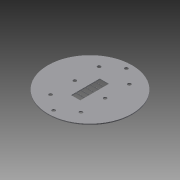
# Autodesk Inventor part: Plate
Saved by Autodesk Inventor 2013 (Build 170138000, 138)
## iProperties
Created: 2014-03-14
Part Number: Plate
Material: Generic
Document SubType Name: Sheet Metal
Designer: jad211
Density: 1 g/cm^3
Sheet Metal Rule: Default_mm
Author: jad211
Autodesk Inventor part; units mm, degrees
ref_plane "YZ Plane" through (0, 0, 0) normal (1, 0, 0) x (0, 1, 0)
ref_plane "XZ Plane" through (0, 0, 0) normal (0, 1, 0) x (-1, 0, 0)
ref_plane "XY Plane" through (0, 0, 0) normal (0, 0, 1) x (1, 0, 0)
sketch "Sketch1" plane through (0, 0, 0) normal (0, 0, 1) x (1, 0, 0)
  circle A0 centre (0, 0) radius 44
  dimension "d0" = 88
  constraints: 1 centre point, 1 coincident
  measures "d0" diameter of A0
extrude "Extrusion1" add sketch "Sketch1" against normal blind 1
sketch "Sketch2" plane through (0, 0, 0) normal (0, 0, 1) x (1, 0, 0)
  circle A0 centre (0, 0) radius 44 projected
  circle A1 centre (0, 38.1) radius 1.75
  circle A2 centre (0, -38.1) radius 1.75
  circle A3 centre (15.87, 0) radius 1.75
  circle A4 centre (-15.88, 0) radius 1.75
  circle A5 centre (-15.87, 25.4) radius 1.75
  circle A6 centre (-15.87, -25.4) radius 1.75
  circle A7 centre (15.87, 25.4) radius 1.75
  circle A8 centre (15.87, -25.4) radius 1.75
  dimension "d4" = 3.5
  dimension "d6" = 3.5
  dimension "d7" = 76.2
  dimension "d8" = 38.1
  dimension "d9" = 3.5
  dimension "d10" = 3.5
  dimension "d11" = 31.75
  dimension "d12" = 15.87
  dimension "d13" = 3.5
  dimension "d14" = 3.5
  dimension "d15" = 3.5
  dimension "d16" = 3.5
  dimension "d17" = 25.4
  dimension "d18" = 25.4
  dimension "d19" = 25.4
  dimension "d20" = 25.4
  dimension "d21" = 15.87
  dimension "d22" = 15.87
  dimension "d23" = 15.87
  dimension "d24" = 15.87
  constraints: 8 centre point
  measures "d4" diameter of A1
  measures "d6" diameter of A2
  measures "d7" distance of A1.centre A2.centre
  measures "d8" distance of A0.centre A2.centre
  measures "d9" diameter of A4
  measures "d10" diameter of A3
  measures "d11" distance of A3.centre A4.centre
  measures "d12" distance of A0.centre A3.centre
  measures "d13" diameter of A7
  measures "d14" diameter of A5
  measures "d15" diameter of A6
  measures "d16" diameter of A8
  measures "d17" distance of A5.centre A4.centre
  measures "d18" distance of A4.centre A6.centre
  measures "d19" distance of A3.centre A8.centre
  measures "d20" distance of A3.centre A7.centre
  measures "d21" horizontal distance of A0.centre A7.centre
  measures "d22" horizontal distance of A0.centre A8.centre
  measures "d23" horizontal distance of A0.centre A6.centre
  measures "d24" horizontal distance of A0.centre A5.centre
hole "Hole2" at (-15.87, 25.4, 0) at (0, 38.1, 0) at (15.87, 25.4, 0) at (15.87, 0, 0) at (15.87, -25.4, 0) at (0, -38.1, 0) at (-15.87, -25.4, 0) at (-15.88, 0, 0) direction (0, 0, -1) diameter 3.5 end through all
sketch "Sketch4" plane through (0, 0, 0) normal (0, 0, 1) x (1, 0, 0)
  circle A0 centre (0, 0) radius 44 projected
  line L0 (-4.7625, 15) -> (4.7625, 15)
  line L1 (4.7625, 15) -> (4.7625, 10.05)
  line L2 (4.7625, 10.05) -> (-4.7625, 10.05)
  line L3 (-4.7625, 10.05) -> (-4.7625, 15)
  line L4 (-4.7625, 9.95) -> (4.7625, 9.95)
  line L5 (4.7625, 9.95) -> (4.7625, 5.05)
  line L6 (4.7625, 5.05) -> (-4.7625, 5.05)
  line L7 (-4.7625, 5.05) -> (-4.7625, 9.95)
  line L8 (-4.7625, 4.95) -> (4.7625, 4.95)
  line L9 (4.7625, 4.95) -> (4.7625, 0.05)
  line L10 (4.7625, 0.05) -> (-4.7625, 0.05)
  line L11 (-4.7625, 0.05) -> (-4.7625, 4.95)
  line L12 (-4.7625, -0.05) -> (4.7625, -0.05)
  line L13 (4.7625, -0.05) -> (4.7625, -4.95)
  line L14 (4.7625, -4.95) -> (-4.7625, -4.95)
  line L15 (-4.7625, -4.95) -> (-4.7625, -0.05)
  line L16 (-4.7625, -5.05) -> (4.7625, -5.05)
  line L17 (4.7625, -5.05) -> (4.7625, -9.95)
  line L18 (4.7625, -9.95) -> (-4.7625, -9.95)
  line L19 (-4.7625, -9.95) -> (-4.7625, -5.05)
  line L20 (-4.7625, -10.05) -> (4.7625, -10.05)
  line L21 (4.7625, -10.05) -> (4.7625, -15)
  line L22 (4.7625, -15) -> (-4.7625, -15)
  line L23 (-4.7625, -15) -> (-4.7625, -10.05)
  dimension "d53" = 9.525
  dimension "d55" = 4.95
  dimension "d56" = 15
  dimension "d57" = 4.7625
  dimension "d58" = 4.9
  dimension "d59" = 9.525
  dimension "d60" = 4.7625
  dimension "d61" = 9.95
  dimension "d62" = 4.9
  dimension "d63" = 0.05
  dimension "d64" = 9.525
  dimension "d65" = 4.7625
  dimension "d66" = 9.525
  dimension "d67" = 4.7625
  dimension "d68" = 4.9
  dimension "d69" = 0.05
  dimension "d70" = 4.9
  dimension "d71" = 9.525
  dimension "d72" = 4.7625
  dimension "d73" = 5.05
  dimension "d74" = 10.05
  dimension "d75" = 4.95
  dimension "d76" = 9.525
  dimension "d77" = 4.7625
  constraints: 48 end point, 12 parallel, 6 horizontal, 6 perpendicular
  measures "d53" distance between parallel lines of L3 L1
  measures "d55" distance between parallel lines of L0 L2
  measures "d56" distance from line of L0 A0.centre
  measures "d57" distance from line of A0.centre L1
  measures "d58" distance between parallel lines of L4 L6
  measures "d59" distance between parallel lines of L7 L5
  measures "d60" distance from line of A0.centre L5
  measures "d61" distance from line of L4 A0.centre
  measures "d62" distance between parallel lines of L8 L10
  measures "d63" distance from line of L10 A0.centre
  measures "d64" distance between parallel lines of L11 L9
  measures "d65" distance from line of A0.centre L9
  measures "d66" distance between parallel lines of L15 L13
  measures "d67" distance from line of A0.centre L13
  measures "d68" distance between parallel lines of L12 L14
  measures "d69" distance from line of L12 A0.centre
  measures "d70" distance between parallel lines of L16 L18
  measures "d71" distance between parallel lines of L19 L17
  measures "d72" distance from line of A0.centre L17
  measures "d73" distance from line of A0.centre L16
  measures "d74" distance from line of A0.centre L20
  measures "d75" distance between parallel lines of L20 L22
  measures "d76" distance between parallel lines of L23 L21
  measures "d77" distance from line of A0.centre L21
extrude "Extrusion2" cut sketch "Sketch4" against normal up to next contours L0 L1 L2 L3 | L4 L5 L6 L7 | L8 L9 L10 L11 | L12 L13 L14 L15 | L16 L17 L18 L19 | L20 L21 L22 L23
equation "\"d6\" = d4"
equation "\"d9\" = d4"
equation "\"d10\" = d4"
equation "\"d13\" = d4"
equation "\"d14\" = d4"
equation "\"d15\" = d4"
equation "\"d16\" = d4"
equation "\"d21\" = d12"
equation "\"d22\" = d12"
equation "\"d23\" = d12"
equation "\"d24\" = d12"
equation "\"d37\" = Thickness"
equation "\"d57\" = 0.5 * d53"
equation "\"d59\" = d53"
equation "\"d60\" = 0.5 * d53"
equation "\"d64\" = d53"
equation "\"d65\" = 0.5 * d53"
equation "\"d66\" = d53"
equation "\"d67\" = 0.5 * d53"
equation "\"d71\" = d53"
equation "\"d72\" = 0.5 * d53"
equation "\"d76\" = d53"
equation "\"d77\" = 0.5 * d53"
equation "\"BendRadius\" = Thickness"
equation "\"BendReliefWidth\" = Thickness"
equation "\"BendReliefDepth\" = 0.5 * Thickness"
equation "\"CornerReliefSize\" = 4 * Thickness"
equation "\"MinimumRemnant\" = 2 * Thickness"
equation "\"TransitionRadius\" = BendRadius"
equation "\"JacobiRadiusSize\" = BendRadius"
equation "\"GapSize\" = Thickness"
equation "\"Thickness\" = 0.5"
body "Solid1"
